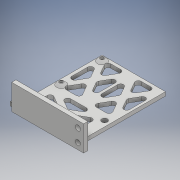
# Autodesk Inventor part: OpenMV&Ping
Saved by Autodesk Inventor 2018 (Build 220112000, 112)
## iProperties
Created: 2018-10-24
Part Number: OpenMV&Ping
Material: 一般
Document SubType Name: Modeling
Designer: shun2
Density: 1 g/cm^3
Appearance: 既定
Author: shun2
Autodesk Inventor part; units mm, degrees
ref_plane "YZ Plane" through (0, 0, 0) normal (1, 0, 0) x (0, 1, 0)
ref_plane "XZ Plane" through (0, 0, 0) normal (0, 1, 0) x (-1, 0, 0)
ref_plane "XY Plane" through (0, 0, 0) normal (0, 0, 1) x (1, 0, 0)
sketch "スケッチ5" plane through (0, 0, 0) normal (0, 0, 1) x (1, 0, 0)
  line L0 (7.2475, 10.0214) -> (7.2475, 21.2492)
  line L1 (-37, -18.3) -> (-36, -17.3)
  line L2 (-37, -18.3) -> (-39, -18.3)
  line L3 (-40, -19.3) -> (-39, -18.3)
  line L4 (-40, -19.3) -> (-40, -23.3)
  circle A0 centre (-35.6, -21.8) radius 2
  circle A1 centre (5.1, -5.5) radius 2
  line L5 (-36, 33.7947) -> (9, 33.7947)
  line L6 (9, 33.7947) -> (9, -24.3)
  line L7 (-36, -17.3) -> (-36, 33.7947)
  arc A2 (2.7155, 28.5133) -> (0.9834, 31.5133) centre (0.9834, 29.5133) ccw
  arc A3 (7.2475, 21.2492) -> (3.5155, 22.2492) centre (5.2475, 21.2492) ccw
  arc A4 (-4.2434, 22.4601) -> (-0.7793, 22.4601) centre (-2.5113, 23.4601) ccw
  line L8 (3.5155, 22.2492) -> (0.2743, 16.6353)
  line L9 (-0.7793, 22.4601) -> (2.7155, 28.5133)
  line L10 (-7.7382, 28.5133) -> (-4.2434, 22.4601)
  arc A5 (-6.0061, 31.5133) -> (-7.7382, 28.5133) centre (-6.0061, 29.5133) ccw
  arc A6 (0.2743, 16.6353) -> (0.2743, 14.6353) centre (2.0064, 15.6353) ccw
  arc A7 (-8.538, 22.2488) -> (-12.27, 21.2488) centre (-10.27, 21.2488) ccw
  line L11 (0.2743, 14.6353) -> (3.5155, 9.0214)
  arc A8 (3.5155, 9.0214) -> (7.2475, 10.0214) centre (5.2475, 10.0214) ccw
  arc A9 (-0.7793, 8.8104) -> (-4.2434, 8.8104) centre (-2.5113, 7.8104) ccw
  line L12 (2.7155, 2.7573) -> (-0.7793, 8.8104)
  arc A10 (0.9834, -0.2427) -> (2.7155, 2.7573) centre (0.9834, 1.7573) ccw
  arc A11 (-25.6467, 22.4601) -> (-22.1826, 22.4601) centre (-23.9146, 23.4601) ccw
  line L13 (-6.0061, -0.2427) -> (0.9834, -0.2427)
  arc A12 (-7.7382, 2.7573) -> (-6.0061, -0.2427) centre (-6.0061, 1.7573) ccw
  line L14 (-14.1558, 10.0214) -> (-14.1558, 21.2492)
  line L15 (-12.27, 21.2488) -> (-12.27, 10.0217)
  line L16 (-5.297, 16.6353) -> (-8.538, 22.2488)
  arc A13 (-12.27, 10.0217) -> (-8.538, 9.0217) centre (-10.27, 10.0217) ccw
  line L17 (-4.2434, 8.8104) -> (-7.7382, 2.7573)
  arc A14 (-5.297, 14.6353) -> (-5.297, 16.6353) centre (-7.029, 15.6353) ccw
  line L18 (-8.538, 9.0217) -> (-5.297, 14.6353)
  line L19 (-22.1826, 22.4601) -> (-18.6878, 28.5133)
  line L20 (-29.1415, 28.5133) -> (-25.6467, 22.4601)
  line L21 (-20.4199, 31.5133) -> (-27.4094, 31.5133)
  arc A15 (-27.4094, 31.5133) -> (-29.1415, 28.5133) centre (-27.4094, 29.5133) ccw
  arc A16 (-18.6878, 28.5133) -> (-20.4199, 31.5133) centre (-20.4199, 29.5133) ccw
  arc A17 (-20.4199, -0.2427) -> (-18.6878, 2.7573) centre (-20.4199, 1.7573) ccw
  line L22 (-17.8878, 22.2492) -> (-21.129, 16.6353)
  line L23 (-21.129, 14.6353) -> (-17.8878, 9.0214)
  line L24 (-18.6878, 2.7573) -> (-22.1826, 8.8104)
  arc A18 (-21.129, 16.6353) -> (-21.129, 14.6353) centre (-19.3969, 15.6353) ccw
  arc A19 (-22.1826, 8.8104) -> (-25.6467, 8.8104) centre (-23.9146, 7.8104) ccw
  line L25 (-27.4094, -0.2427) -> (-20.4199, -0.2427)
  arc A20 (-29.1415, 2.7573) -> (-27.4094, -0.2427) centre (-27.4094, 1.7573) ccw
  line L26 (-25.6467, 8.8104) -> (-29.1415, 2.7573)
  arc A21 (-26.7003, 14.6353) -> (-26.7003, 16.6353) centre (-28.4323, 15.6353) ccw
  line L27 (-29.9413, 9.0217) -> (-26.7003, 14.6353)
  line L28 (-26.7003, 16.6353) -> (-29.9413, 22.2488)
  arc A22 (-33.6733, 10.0217) -> (-29.9413, 9.0217) centre (-31.6733, 10.0217) ccw
  line L29 (-33.6733, 21.2488) -> (-33.6733, 10.0217)
  arc A23 (-29.9413, 22.2488) -> (-33.6733, 21.2488) centre (-31.6733, 21.2488) ccw
  arc A24 (-17.8878, 9.0214) -> (-14.1558, 10.0214) centre (-16.1558, 10.0214) ccw
  arc A25 (-14.1558, 21.2492) -> (-17.8878, 22.2492) centre (-16.1558, 21.2492) ccw
  line L30 (0.9834, 31.5133) -> (-6.0061, 31.5133)
  line L31 (-40, -24.3) -> (-40, -27.3)
  line L32 (-40, -27.3) -> (9, -27.3)
  line L33 (9, -27.3) -> (9, -24.3)
  line L34 (-40, -23.3) -> (-40, -24.3)
  line L35 (-9.1215, -4.2017) -> (-20.3493, -4.2017)
  arc A26 (-27.6134, -8.7338) -> (-30.6134, -10.4658) centre (-28.6134, -10.4658) ccw
  arc A27 (-21.5603, -15.6926) -> (-21.5603, -12.2285) centre (-22.5603, -13.9606) ccw
  line L36 (-21.5603, -12.2285) -> (-27.6134, -8.7338)
  line L37 (-27.6134, -19.1874) -> (-21.5603, -15.6926)
  line L38 (-30.6134, -10.4658) -> (-30.6134, -17.4554)
  arc A28 (-30.6134, -17.4554) -> (-27.6134, -19.1874) centre (-28.6134, -17.4554) ccw
  line L39 (-13.7354, -11.1749) -> (-8.1215, -7.9338)
  arc A29 (-7.9105, -12.2285) -> (-7.9105, -15.6926) centre (-6.9105, -13.9606) ccw
  arc A30 (-9.1218, -23.7193) -> (-8.1218, -19.9872) centre (-9.1218, -21.7193) ccw
  line L40 (1.1426, -17.4554) -> (1.1426, -10.4658)
  arc A31 (1.1426, -10.4658) -> (-1.8574, -8.7338) centre (-0.8574, -10.4658) ccw
  arc A32 (-20.3493, -4.2017) -> (-21.3493, -7.9338) centre (-20.3493, -6.2017) ccw
  arc A33 (-21.3489, -19.9872) -> (-20.3489, -23.7193) centre (-20.3489, -21.7193) ccw
  line L41 (-21.3493, -7.9338) -> (-15.7354, -11.1749)
  line L42 (-15.7354, -16.7462) -> (-21.3489, -19.9872)
  arc A34 (-15.7354, -11.1749) -> (-13.7354, -11.1749) centre (-14.7354, -9.4429) ccw
  arc A35 (-13.7354, -16.7462) -> (-15.7354, -16.7462) centre (-14.7354, -18.4783) ccw
  line L43 (-20.3489, -23.7193) -> (-9.1218, -23.7193)
  line L44 (-8.1218, -19.9872) -> (-13.7354, -16.7462)
  arc A36 (-8.1215, -7.9338) -> (-9.1215, -4.2017) centre (-9.1215, -6.2017) ccw
  line L45 (-1.8574, -8.7338) -> (-7.9105, -12.2285)
  line L46 (-7.9105, -15.6926) -> (-1.8574, -19.1874)
  arc A37 (-1.8574, -19.1874) -> (1.1426, -17.4554) centre (-0.8574, -17.4554) ccw
  circle A38 centre (-32.2733, 30.1133) radius 1.1
  circle A39 centre (-32.2733, 1.1573) radius 1.1
  dimension "d11" = 45
  dimension "d12" = 2.2
  dimension "d13" = 2.2
  constraints: 94 end point, 72 point on circle, 40 centre point, 2 parallel, 1 collinear
  measures "d11" distance of L5.start L5.end
  measures "d12" diameter of A38
  measures "d13" diameter of A39
extrude "押し出し2" add sketch "スケッチ5" along normal blind 2.7
sketch "スケッチ8" plane through (0, 0, 0) normal (0, 0, -1) x (-1, 0, 0)
  line L0 (-15, -27.3) -> (36, -27.3)
  line L1 (36, -27.3) -> (36, -30.3)
  line L2 (36, -30.3) -> (-15, -30.3)
  line L3 (-15, -30.3) -> (-15, -27.3)
  arc A0 (9.1215, -4.2017) -> (8.1215, -7.9338) centre (9.1215, -6.2017) ccw projected
  line L4 (9.1215, -4.2017) -> (20.3493, -4.2017) projected
  arc A1 (21.3493, -7.9338) -> (20.3493, -4.2017) centre (20.3493, -6.2017) ccw projected
  line L5 (21.3493, -7.9338) -> (15.7354, -11.1749) projected
  arc A2 (13.7354, -11.1749) -> (15.7354, -11.1749) centre (14.7354, -9.4429) ccw projected
  line L6 (13.7354, -11.1749) -> (8.1215, -7.9338) projected
  arc A3 (17.8878, 22.2492) -> (14.1558, 21.2492) centre (16.1558, 21.2492) ccw projected
  line L7 (17.8878, 22.2492) -> (21.129, 16.6353) projected
  arc A4 (21.129, 14.6353) -> (21.129, 16.6353) centre (19.3969, 15.6353) ccw projected
  line L8 (21.129, 14.6353) -> (17.8878, 9.0214) projected
  arc A5 (14.1558, 10.0214) -> (17.8878, 9.0214) centre (16.1558, 10.0214) ccw projected
  line L9 (14.1558, 10.0214) -> (14.1558, 21.2492) projected
  arc A6 (-7.2475, 10.0214) -> (-3.5155, 9.0214) centre (-5.2475, 10.0214) ccw projected
  line L10 (-7.2475, 10.0214) -> (-7.2475, 21.2492) projected
  arc A7 (-3.5155, 22.2492) -> (-7.2475, 21.2492) centre (-5.2475, 21.2492) ccw projected
  line L11 (-3.5155, 22.2492) -> (-0.2743, 16.6353) projected
  arc A8 (-0.2743, 14.6353) -> (-0.2743, 16.6353) centre (-2.0064, 15.6353) ccw projected
  line L12 (-0.2743, 14.6353) -> (-3.5155, 9.0214) projected
  arc A9 (15.7354, -16.7462) -> (13.7354, -16.7462) centre (14.7354, -18.4783) ccw projected
  line L13 (15.7354, -16.7462) -> (21.3489, -19.9872) projected
  arc A10 (20.3489, -23.7193) -> (21.3489, -19.9872) centre (20.3489, -21.7193) ccw projected
  line L14 (20.3489, -23.7193) -> (9.1218, -23.7193) projected
  arc A11 (8.1218, -19.9872) -> (9.1218, -23.7193) centre (9.1218, -21.7193) ccw projected
  line L15 (8.1218, -19.9872) -> (13.7354, -16.7462) projected
  arc A12 (33.6733, 21.2488) -> (29.9413, 22.2488) centre (31.6733, 21.2488) ccw projected
  line L16 (33.6733, 21.2488) -> (33.6733, 10.0217) projected
  arc A13 (29.9413, 9.0217) -> (33.6733, 10.0217) centre (31.6733, 10.0217) ccw projected
  line L17 (29.9413, 9.0217) -> (26.7003, 14.6353) projected
  arc A14 (26.7003, 16.6353) -> (26.7003, 14.6353) centre (28.4323, 15.6353) ccw projected
  line L18 (26.7003, 16.6353) -> (29.9413, 22.2488) projected
  line L19 (8.538, 9.0217) -> (5.297, 14.6353) projected
  arc A15 (5.297, 16.6353) -> (5.297, 14.6353) centre (7.029, 15.6353) ccw projected
  line L20 (5.297, 16.6353) -> (8.538, 22.2488) projected
  arc A16 (12.27, 21.2488) -> (8.538, 22.2488) centre (10.27, 21.2488) ccw projected
  line L21 (12.27, 21.2488) -> (12.27, 10.0217) projected
  arc A17 (8.538, 9.0217) -> (12.27, 10.0217) centre (10.27, 10.0217) ccw projected
  arc A18 (1.8574, -8.7338) -> (-1.1426, -10.4658) centre (0.8574, -10.4658) ccw projected
  line L22 (1.8574, -8.7338) -> (7.9105, -12.2285) projected
  arc A19 (7.9105, -15.6926) -> (7.9105, -12.2285) centre (6.9105, -13.9606) ccw projected
  line L23 (7.9105, -15.6926) -> (1.8574, -19.1874) projected
  arc A20 (-1.1426, -17.4554) -> (1.8574, -19.1874) centre (0.8574, -17.4554) ccw projected
  line L24 (-1.1426, -17.4554) -> (-1.1426, -10.4658) projected
  arc A21 (27.6134, -19.1874) -> (30.6134, -17.4554) centre (28.6134, -17.4554) ccw projected
  line L25 (27.6134, -19.1874) -> (21.5603, -15.6926) projected
  arc A22 (21.5603, -12.2285) -> (21.5603, -15.6926) centre (22.5603, -13.9606) ccw projected
  line L26 (21.5603, -12.2285) -> (27.6134, -8.7338) projected
  arc A23 (30.6134, -10.4658) -> (27.6134, -8.7338) centre (28.6134, -10.4658) ccw projected
  line L27 (30.6134, -10.4658) -> (30.6134, -17.4554) projected
  arc A24 (29.1415, 28.5133) -> (27.4094, 31.5133) centre (27.4094, 29.5133) ccw projected
  line L28 (29.1415, 28.5133) -> (25.6467, 22.4601) projected
  arc A25 (22.1826, 22.4601) -> (25.6467, 22.4601) centre (23.9146, 23.4601) ccw projected
  line L29 (22.1826, 22.4601) -> (18.6878, 28.5133) projected
  arc A26 (20.4199, 31.5133) -> (18.6878, 28.5133) centre (20.4199, 29.5133) ccw projected
  line L30 (20.4199, 31.5133) -> (27.4094, 31.5133) projected
  line L31 (18.6878, 2.7573) -> (22.1826, 8.8104) projected
  arc A27 (25.6467, 8.8104) -> (22.1826, 8.8104) centre (23.9146, 7.8104) ccw projected
  line L32 (25.6467, 8.8104) -> (29.1415, 2.7573) projected
  arc A28 (27.4094, -0.2427) -> (29.1415, 2.7573) centre (27.4094, 1.7573) ccw projected
  line L33 (27.4094, -0.2427) -> (20.4199, -0.2427) projected
  arc A29 (18.6878, 2.7573) -> (20.4199, -0.2427) centre (20.4199, 1.7573) ccw projected
  arc A30 (-2.7155, 2.7573) -> (-0.9834, -0.2427) centre (-0.9834, 1.7573) ccw projected
  line L34 (-2.7155, 2.7573) -> (0.7793, 8.8104) projected
  arc A31 (4.2434, 8.8104) -> (0.7793, 8.8104) centre (2.5113, 7.8104) ccw projected
  line L35 (4.2434, 8.8104) -> (7.7382, 2.7573) projected
  arc A32 (6.0061, -0.2427) -> (7.7382, 2.7573) centre (6.0061, 1.7573) ccw projected
  line L36 (6.0061, -0.2427) -> (-0.9834, -0.2427) projected
  line L37 (0.7793, 22.4601) -> (-2.7155, 28.5133) projected
  arc A33 (-0.9834, 31.5133) -> (-2.7155, 28.5133) centre (-0.9834, 29.5133) ccw projected
  line L38 (-0.9834, 31.5133) -> (6.0061, 31.5133) projected
  arc A34 (7.7382, 28.5133) -> (6.0061, 31.5133) centre (6.0061, 29.5133) ccw projected
  line L39 (7.7382, 28.5133) -> (4.2434, 22.4601) projected
  arc A35 (0.7793, 22.4601) -> (4.2434, 22.4601) centre (2.5113, 23.4601) ccw projected
  circle A36 centre (35.6, -21.8) radius 2 projected
  circle A37 centre (-5.1, -5.5) radius 2 projected
  circle A38 centre (32.2733, 30.1133) radius 1.1 projected
  circle A39 centre (32.2733, 1.1573) radius 1.1 projected
  line L40 (37, -18.3) -> (36, -17.3) projected
  line L41 (36, -17.3) -> (36, 33.7947) projected
  line L42 (36, 33.7947) -> (-9, 33.7947) projected
  line L43 (-9, 33.7947) -> (-9, -27.3) projected
  line L44 (-9, -27.3) -> (40, -27.3) projected
  line L45 (40, -27.3) -> (40, -19.3) projected
  line L46 (40, -19.3) -> (39, -18.3) projected
  line L47 (39, -18.3) -> (37, -18.3) projected
  line L48 (36, -30.3) -> (36, -27.3) projected
  point P0 (0, 0)
  dimension "d19" = 51
  dimension "d20" = 3
  constraints: 8 end point, 2 parallel, 1 horizontal, 1 perpendicular
  measures "d19" distance of L2.start L3.start
  measures "d20" distance of L1.start L2.start
extrude "押し出し3" add sketch "スケッチ8" against normal blind 18 contours L0 L1 L2 L3
sketch "スケッチ9" plane through (9, -27.3, 0) normal (0, 1, 0) x (1, 0, 0)
  circle A0 centre (2, -4.5) radius 1.8
  line L0 (0, 0) -> (6, 0) projected
  line L1 (6, 0) -> (6, -18) projected
  circle A1 centre (2, -13.5) radius 1.8
  point P0 (-9, 0)
  dimension "d23" = 3.6
  dimension "d24" = 4.5
  dimension "d25" = 4
  dimension "d26" = 3.6
  dimension "d27" = 13.5
  dimension "d28" = 4
  constraints: 2 centre point
  measures "d23" diameter of A0
  measures "d24" distance from line of L0 A0.centre
  measures "d25" distance from line of L1 A0.centre
  measures "d26" diameter of A1
  measures "d27" distance from line of L0 A1.centre
  measures "d28" distance from line of L1 A1.centre
extrude "押し出し4" cut sketch "スケッチ9" against normal blind 3
chamfer "面取り1" distance 1 angle 45 2 edges at (9, -27.3, 1.35) (-13.5, -27.3, 2.7)
sketch "スケッチ10" plane through (0, 0, 2.7) normal (0, 0, 1) x (1, 0, 0)
  line L0 (9, -26.3) -> (-36, -26.3) projected
  line L1 (9, -26.3) -> (9, 33.7947) projected
  line L2 (9, 33.7947) -> (-36, 33.7947) projected
  line L3 (-36, 33.7947) -> (-36, -17.3) projected
  line L4 (-36, -17.3) -> (-37, -18.3) projected
  line L5 (-37, -18.3) -> (-39, -18.3) projected
  line L6 (-39, -18.3) -> (-40, -19.3) projected
  line L7 (-40, -19.3) -> (-40, -27.3) projected
  line L8 (-40, -27.3) -> (-36, -27.3) projected
  line L9 (-36, -27.3) -> (-36, -26.3) projected
  arc A0 (-8.1215, -7.9338) -> (-9.1215, -4.2017) centre (-9.1215, -6.2017) ccw projected
  line L10 (-8.1215, -7.9338) -> (-13.7354, -11.1749) projected
  arc A1 (-15.7354, -11.1749) -> (-13.7354, -11.1749) centre (-14.7354, -9.4429) ccw projected
  line L11 (-15.7354, -11.1749) -> (-21.3493, -7.9338) projected
  arc A2 (-20.3493, -4.2017) -> (-21.3493, -7.9338) centre (-20.3493, -6.2017) ccw projected
  line L12 (-20.3493, -4.2017) -> (-9.1215, -4.2017) projected
  arc A3 (-14.1558, 21.2492) -> (-17.8878, 22.2492) centre (-16.1558, 21.2492) ccw projected
  line L13 (-14.1558, 21.2492) -> (-14.1558, 10.0214) projected
  arc A4 (-17.8878, 9.0214) -> (-14.1558, 10.0214) centre (-16.1558, 10.0214) ccw projected
  line L14 (-17.8878, 9.0214) -> (-21.129, 14.6353) projected
  arc A5 (-21.129, 16.6353) -> (-21.129, 14.6353) centre (-19.3969, 15.6353) ccw projected
  line L15 (-21.129, 16.6353) -> (-17.8878, 22.2492) projected
  arc A6 (3.5155, 9.0214) -> (7.2475, 10.0214) centre (5.2475, 10.0214) ccw projected
  line L16 (3.5155, 9.0214) -> (0.2743, 14.6353) projected
  arc A7 (0.2743, 16.6353) -> (0.2743, 14.6353) centre (2.0064, 15.6353) ccw projected
  line L17 (0.2743, 16.6353) -> (3.5155, 22.2492) projected
  arc A8 (7.2475, 21.2492) -> (3.5155, 22.2492) centre (5.2475, 21.2492) ccw projected
  line L18 (7.2475, 21.2492) -> (7.2475, 10.0214) projected
  arc A9 (-13.7354, -16.7462) -> (-15.7354, -16.7462) centre (-14.7354, -18.4783) ccw projected
  line L19 (-13.7354, -16.7462) -> (-8.1218, -19.9872) projected
  arc A10 (-9.1218, -23.7193) -> (-8.1218, -19.9872) centre (-9.1218, -21.7193) ccw projected
  line L20 (-9.1218, -23.7193) -> (-20.3489, -23.7193) projected
  arc A11 (-21.3489, -19.9872) -> (-20.3489, -23.7193) centre (-20.3489, -21.7193) ccw projected
  line L21 (-21.3489, -19.9872) -> (-15.7354, -16.7462) projected
  arc A12 (-29.9413, 22.2488) -> (-33.6733, 21.2488) centre (-31.6733, 21.2488) ccw projected
  line L22 (-29.9413, 22.2488) -> (-26.7003, 16.6353) projected
  arc A13 (-26.7003, 14.6353) -> (-26.7003, 16.6353) centre (-28.4323, 15.6353) ccw projected
  line L23 (-26.7003, 14.6353) -> (-29.9413, 9.0217) projected
  arc A14 (-33.6733, 10.0217) -> (-29.9413, 9.0217) centre (-31.6733, 10.0217) ccw projected
  line L24 (-33.6733, 10.0217) -> (-33.6733, 21.2488) projected
  line L25 (-5.297, 14.6353) -> (-8.538, 9.0217) projected
  arc A15 (-12.27, 10.0217) -> (-8.538, 9.0217) centre (-10.27, 10.0217) ccw projected
  line L26 (-12.27, 10.0217) -> (-12.27, 21.2488) projected
  arc A16 (-8.538, 22.2488) -> (-12.27, 21.2488) centre (-10.27, 21.2488) ccw projected
  line L27 (-8.538, 22.2488) -> (-5.297, 16.6353) projected
  arc A17 (-5.297, 14.6353) -> (-5.297, 16.6353) centre (-7.029, 15.6353) ccw projected
  arc A18 (1.1426, -10.4658) -> (-1.8574, -8.7338) centre (-0.8574, -10.4658) ccw projected
  line L28 (1.1426, -10.4658) -> (1.1426, -17.4554) projected
  arc A19 (-1.8574, -19.1874) -> (1.1426, -17.4554) centre (-0.8574, -17.4554) ccw projected
  line L29 (-1.8574, -19.1874) -> (-7.9105, -15.6926) projected
  arc A20 (-7.9105, -12.2285) -> (-7.9105, -15.6926) centre (-6.9105, -13.9606) ccw projected
  line L30 (-7.9105, -12.2285) -> (-1.8574, -8.7338) projected
  arc A21 (-30.6134, -17.4554) -> (-27.6134, -19.1874) centre (-28.6134, -17.4554) ccw projected
  line L31 (-30.6134, -17.4554) -> (-30.6134, -10.4658) projected
  arc A22 (-27.6134, -8.7338) -> (-30.6134, -10.4658) centre (-28.6134, -10.4658) ccw projected
  line L32 (-27.6134, -8.7338) -> (-21.5603, -12.2285) projected
  arc A23 (-21.5603, -15.6926) -> (-21.5603, -12.2285) centre (-22.5603, -13.9606) ccw projected
  line L33 (-21.5603, -15.6926) -> (-27.6134, -19.1874) projected
  arc A24 (-27.4094, 31.5133) -> (-29.1415, 28.5133) centre (-27.4094, 29.5133) ccw projected
  line L34 (-27.4094, 31.5133) -> (-20.4199, 31.5133) projected
  arc A25 (-18.6878, 28.5133) -> (-20.4199, 31.5133) centre (-20.4199, 29.5133) ccw projected
  line L35 (-18.6878, 28.5133) -> (-22.1826, 22.4601) projected
  arc A26 (-25.6467, 22.4601) -> (-22.1826, 22.4601) centre (-23.9146, 23.4601) ccw projected
  line L36 (-25.6467, 22.4601) -> (-29.1415, 28.5133) projected
  line L37 (-22.1826, 8.8104) -> (-18.6878, 2.7573) projected
  arc A27 (-20.4199, -0.2427) -> (-18.6878, 2.7573) centre (-20.4199, 1.7573) ccw projected
  line L38 (-20.4199, -0.2427) -> (-27.4094, -0.2427) projected
  arc A28 (-29.1415, 2.7573) -> (-27.4094, -0.2427) centre (-27.4094, 1.7573) ccw projected
  line L39 (-29.1415, 2.7573) -> (-25.6467, 8.8104) projected
  arc A29 (-22.1826, 8.8104) -> (-25.6467, 8.8104) centre (-23.9146, 7.8104) ccw projected
  arc A30 (0.9834, -0.2427) -> (2.7155, 2.7573) centre (0.9834, 1.7573) ccw projected
  line L40 (0.9834, -0.2427) -> (-6.0061, -0.2427) projected
  arc A31 (-7.7382, 2.7573) -> (-6.0061, -0.2427) centre (-6.0061, 1.7573) ccw projected
  line L41 (-7.7382, 2.7573) -> (-4.2434, 8.8104) projected
  arc A32 (-0.7793, 8.8104) -> (-4.2434, 8.8104) centre (-2.5113, 7.8104) ccw projected
  line L42 (-0.7793, 8.8104) -> (2.7155, 2.7573) projected
  line L43 (2.7155, 28.5133) -> (-0.7793, 22.4601) projected
  arc A33 (-4.2434, 22.4601) -> (-0.7793, 22.4601) centre (-2.5113, 23.4601) ccw projected
  line L44 (-4.2434, 22.4601) -> (-7.7382, 28.5133) projected
  arc A34 (-6.0061, 31.5133) -> (-7.7382, 28.5133) centre (-6.0061, 29.5133) ccw projected
  line L45 (-6.0061, 31.5133) -> (0.9834, 31.5133) projected
  arc A35 (2.7155, 28.5133) -> (0.9834, 31.5133) centre (0.9834, 29.5133) ccw projected
  circle A36 centre (-35.6, -21.8) radius 2 projected
  circle A37 centre (5.1, -5.5) radius 2 projected
  circle A38 centre (-32.2733, 30.1133) radius 1.1 projected
  circle A39 centre (-32.2733, 1.1573) radius 1.1 projected
  circle A40 centre (-32.2733, 30.1133) radius 1.5
  circle A41 centre (-32.2733, 1.1573) radius 1.5
  point P0 (0, 0)
  dimension "d34" = 3
  dimension "d35" = 3
  constraints: 2 centre point, 2 coincident
  measures "d34" diameter of A40
  measures "d35" diameter of A41
extrude "押し出し5" add sketch "スケッチ10" along normal blind 1.8 contours A40 | A41
chamfer "面取り2" distance 1.8 angle 45 2 edges at (-33.7733, 30.1133, 2.7) (-33.7733, 1.1573, 2.7)
sketch "スケッチ11" plane through (0, 0, 0) normal (0, 0, -1) x (-1, 0, 0)
  arc A0 (9.1215, -4.2017) -> (8.1215, -7.9338) centre (9.1215, -6.2017) ccw projected
  line L0 (9.1215, -4.2017) -> (20.3493, -4.2017) projected
  arc A1 (21.3493, -7.9338) -> (20.3493, -4.2017) centre (20.3493, -6.2017) ccw projected
  line L1 (21.3493, -7.9338) -> (15.7354, -11.1749) projected
  arc A2 (13.7354, -11.1749) -> (15.7354, -11.1749) centre (14.7354, -9.4429) ccw projected
  line L2 (13.7354, -11.1749) -> (8.1215, -7.9338) projected
  arc A3 (17.8878, 22.2492) -> (14.1558, 21.2492) centre (16.1558, 21.2492) ccw projected
  line L3 (17.8878, 22.2492) -> (21.129, 16.6353) projected
  arc A4 (21.129, 14.6353) -> (21.129, 16.6353) centre (19.3969, 15.6353) ccw projected
  line L4 (21.129, 14.6353) -> (17.8878, 9.0214) projected
  arc A5 (14.1558, 10.0214) -> (17.8878, 9.0214) centre (16.1558, 10.0214) ccw projected
  line L5 (14.1558, 10.0214) -> (14.1558, 21.2492) projected
  arc A6 (-7.2475, 10.0214) -> (-3.5155, 9.0214) centre (-5.2475, 10.0214) ccw projected
  line L6 (-7.2475, 10.0214) -> (-7.2475, 21.2492) projected
  arc A7 (-3.5155, 22.2492) -> (-7.2475, 21.2492) centre (-5.2475, 21.2492) ccw projected
  line L7 (-3.5155, 22.2492) -> (-0.2743, 16.6353) projected
  arc A8 (-0.2743, 14.6353) -> (-0.2743, 16.6353) centre (-2.0064, 15.6353) ccw projected
  line L8 (-0.2743, 14.6353) -> (-3.5155, 9.0214) projected
  arc A9 (15.7354, -16.7462) -> (13.7354, -16.7462) centre (14.7354, -18.4783) ccw projected
  line L9 (15.7354, -16.7462) -> (21.3489, -19.9872) projected
  arc A10 (20.3489, -23.7193) -> (21.3489, -19.9872) centre (20.3489, -21.7193) ccw projected
  line L10 (20.3489, -23.7193) -> (9.1218, -23.7193) projected
  arc A11 (8.1218, -19.9872) -> (9.1218, -23.7193) centre (9.1218, -21.7193) ccw projected
  line L11 (8.1218, -19.9872) -> (13.7354, -16.7462) projected
  arc A12 (33.6733, 21.2488) -> (29.9413, 22.2488) centre (31.6733, 21.2488) ccw projected
  line L12 (33.6733, 21.2488) -> (33.6733, 10.0217) projected
  arc A13 (29.9413, 9.0217) -> (33.6733, 10.0217) centre (31.6733, 10.0217) ccw projected
  line L13 (29.9413, 9.0217) -> (26.7003, 14.6353) projected
  arc A14 (26.7003, 16.6353) -> (26.7003, 14.6353) centre (28.4323, 15.6353) ccw projected
  line L14 (26.7003, 16.6353) -> (29.9413, 22.2488) projected
  line L15 (8.538, 9.0217) -> (5.297, 14.6353) projected
  arc A15 (5.297, 16.6353) -> (5.297, 14.6353) centre (7.029, 15.6353) ccw projected
  line L16 (5.297, 16.6353) -> (8.538, 22.2488) projected
  arc A16 (12.27, 21.2488) -> (8.538, 22.2488) centre (10.27, 21.2488) ccw projected
  line L17 (12.27, 21.2488) -> (12.27, 10.0217) projected
  arc A17 (8.538, 9.0217) -> (12.27, 10.0217) centre (10.27, 10.0217) ccw projected
  arc A18 (1.8574, -8.7338) -> (-1.1426, -10.4658) centre (0.8574, -10.4658) ccw projected
  line L18 (1.8574, -8.7338) -> (7.9105, -12.2285) projected
  arc A19 (7.9105, -15.6926) -> (7.9105, -12.2285) centre (6.9105, -13.9606) ccw projected
  line L19 (7.9105, -15.6926) -> (1.8574, -19.1874) projected
  arc A20 (-1.1426, -17.4554) -> (1.8574, -19.1874) centre (0.8574, -17.4554) ccw projected
  line L20 (-1.1426, -17.4554) -> (-1.1426, -10.4658) projected
  arc A21 (27.6134, -19.1874) -> (30.6134, -17.4554) centre (28.6134, -17.4554) ccw projected
  line L21 (27.6134, -19.1874) -> (21.5603, -15.6926) projected
  arc A22 (21.5603, -12.2285) -> (21.5603, -15.6926) centre (22.5603, -13.9606) ccw projected
  line L22 (21.5603, -12.2285) -> (27.6134, -8.7338) projected
  arc A23 (30.6134, -10.4658) -> (27.6134, -8.7338) centre (28.6134, -10.4658) ccw projected
  line L23 (30.6134, -10.4658) -> (30.6134, -17.4554) projected
  arc A24 (29.1415, 28.5133) -> (27.4094, 31.5133) centre (27.4094, 29.5133) ccw projected
  line L24 (29.1415, 28.5133) -> (25.6467, 22.4601) projected
  arc A25 (22.1826, 22.4601) -> (25.6467, 22.4601) centre (23.9146, 23.4601) ccw projected
  line L25 (22.1826, 22.4601) -> (18.6878, 28.5133) projected
  arc A26 (20.4199, 31.5133) -> (18.6878, 28.5133) centre (20.4199, 29.5133) ccw projected
  line L26 (20.4199, 31.5133) -> (27.4094, 31.5133) projected
  line L27 (18.6878, 2.7573) -> (22.1826, 8.8104) projected
  arc A27 (25.6467, 8.8104) -> (22.1826, 8.8104) centre (23.9146, 7.8104) ccw projected
  line L28 (25.6467, 8.8104) -> (29.1415, 2.7573) projected
  arc A28 (27.4094, -0.2427) -> (29.1415, 2.7573) centre (27.4094, 1.7573) ccw projected
  line L29 (27.4094, -0.2427) -> (20.4199, -0.2427) projected
  arc A29 (18.6878, 2.7573) -> (20.4199, -0.2427) centre (20.4199, 1.7573) ccw projected
  arc A30 (-2.7155, 2.7573) -> (-0.9834, -0.2427) centre (-0.9834, 1.7573) ccw projected
  line L30 (-2.7155, 2.7573) -> (0.7793, 8.8104) projected
  arc A31 (4.2434, 8.8104) -> (0.7793, 8.8104) centre (2.5113, 7.8104) ccw projected
  line L31 (4.2434, 8.8104) -> (7.7382, 2.7573) projected
  arc A32 (6.0061, -0.2427) -> (7.7382, 2.7573) centre (6.0061, 1.7573) ccw projected
  line L32 (6.0061, -0.2427) -> (-0.9834, -0.2427) projected
  line L33 (0.7793, 22.4601) -> (-2.7155, 28.5133) projected
  arc A33 (-0.9834, 31.5133) -> (-2.7155, 28.5133) centre (-0.9834, 29.5133) ccw projected
  line L34 (-0.9834, 31.5133) -> (6.0061, 31.5133) projected
  arc A34 (7.7382, 28.5133) -> (6.0061, 31.5133) centre (6.0061, 29.5133) ccw projected
  line L35 (7.7382, 28.5133) -> (4.2434, 22.4601) projected
  arc A35 (0.7793, 22.4601) -> (4.2434, 22.4601) centre (2.5113, 23.4601) ccw projected
  circle A36 centre (35.6, -21.8) radius 2 projected
  circle A37 centre (-5.1, -5.5) radius 2 projected
  circle A38 centre (32.2733, 30.1133) radius 1.1 projected
  circle A39 centre (32.2733, 1.1573) radius 1.1 projected
  line L36 (37, -18.3) -> (36, -17.3) projected
  line L37 (36, -17.3) -> (36, 33.7947) projected
  line L38 (36, 33.7947) -> (-9, 33.7947) projected
  line L39 (-9, 33.7947) -> (-9, -26.3) projected
  line L40 (-10, -27.3) -> (-9, -26.3) projected
  line L41 (-10, -27.3) -> (-15, -27.3) projected
  line L42 (-15, -27.3) -> (-15, -30.3) projected
  line L43 (-15, -30.3) -> (36, -30.3) projected
  line L44 (36, -30.3) -> (36, -27.3) projected
  line L45 (36, -27.3) -> (40, -27.3) projected
  line L46 (40, -27.3) -> (40, -19.3) projected
  line L47 (40, -19.3) -> (39, -18.3) projected
  line L48 (39, -18.3) -> (37, -18.3) projected
  line L49 (34.0952, 0.1547) -> (32.316, -0.9218)
  line L50 (32.316, -0.9218) -> (30.4941, 0.0808)
  line L51 (30.4941, 0.0808) -> (30.4515, 2.1599)
  line L52 (30.4515, 2.1599) -> (32.2307, 3.2363)
  line L53 (32.2307, 3.2363) -> (34.0525, 2.2338)
  line L54 (34.0525, 2.2338) -> (34.0952, 0.1547)
  line L55 (34.0952, 29.1107) -> (32.316, 28.0342)
  line L56 (32.316, 28.0342) -> (30.4941, 29.0368)
  line L57 (30.4941, 29.0368) -> (30.4515, 31.1159)
  line L58 (30.4515, 31.1159) -> (32.2307, 32.1923)
  line L59 (32.2307, 32.1923) -> (34.0525, 31.1898)
  line L60 (34.0525, 31.1898) -> (34.0952, 29.1107)
  point P0 (0, 0)
  constraints: 24 end point, 1 coincident, 26 other
extrude "押し出し6" cut sketch "スケッチ11" against normal blind 1.5 contours L49 L50 L51 L52 L53 L54 | L55 L56 L57 L58 L59 L60
